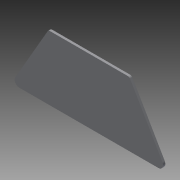
# Autodesk Inventor part: Chair Support Side
Saved by Autodesk Inventor 2015 (Build 190159000, 159)
## iProperties
Created: 2016-03-22
Part Number: Chair Support Side
Material: Generic
Document SubType Name: Modeling
Designer: Mac
Density: 1 g/cm^3
Appearance: Default
Author: Mac
Autodesk Inventor part; units mm, degrees
ref_plane "YZ Plane" through (0, 0, 0) normal (1, 0, 0) x (0, 1, 0)
ref_plane "XZ Plane" through (0, 0, 0) normal (0, 1, 0) x (-1, 0, 0)
ref_plane "XY Plane" through (0, 0, 0) normal (0, 0, 1) x (1, 0, 0)
sketch "Sketch1" plane through (0, 0, 0) normal (0, 0, 1) x (1, 0, 0)
  line L0 (-289.9677, -132.6403) -> (218.0323, -132.6403)
  line L1 (230.2995, -116.6532) -> (167.7853, 116.6532)
  line L2 (-300.9662, -113.5903) -> (-167.1509, 118.1847)
  line L3 (-311.9648, -132.6403) -> (-44.334, -132.6403) construction
  line L4 (-161.6516, 121.3597) -> (161.6516, 121.3597)
  arc A0 (167.7853, 116.6532) -> (161.6516, 121.3597) centre (161.6516, 115.0097) ccw
  arc A1 (-161.6516, 121.3597) -> (-167.1509, 118.1847) centre (-161.6516, 115.0097) ccw
  arc A2 (-300.9662, -113.5903) -> (-289.9677, -132.6403) centre (-289.9677, -119.9403) ccw
  arc A3 (218.0323, -132.6403) -> (230.2995, -116.6532) centre (218.0323, -119.9403) ccw
  point P0 (0, 0)
  point P1 (0, 121.3597)
  point P2 (199.0424, 0)
  dimension "d0" = 75
  dimension "d1" = 60
  dimension "d2" = 6.35
  dimension "d3" = 6.35
  dimension "d4" = 12.7
  dimension "d5" = 508
  dimension "d11" = 254
  constraints: 10 end point, 8 point on circle, 8 tangent, 4 centre point, 3 horizontal, 2 midpoint, 2 point on line, 1 equal length, 1 equal radius, 1 horizontal alignment, 1 vertical alignment
  measures "d0" angle of L1 L0
  measures "d1" angle of L3 L2
  measures "d2" radius of A0
  measures "d3" radius of A1
  measures "d4" radius of A2
  measures "d5" distance of L0.start L0.end
  measures "d11" distance between parallel lines of L0 L4
extrude "Extrusion1" add sketch "Sketch1" along normal blind 6.35
body "Solid1"
